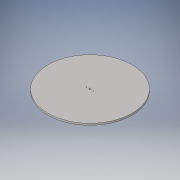
# Autodesk Inventor part: Zoetrope_Top
Saved by Autodesk Inventor 2016 (Build 200138000, 138)
## iProperties
Created: 2019-02-14
Part Number: Zoetrope_Top
Material: Generic
Document SubType Name: Modeling
Designer: student
Density: 1 g/cm^3
Appearance: Default
Author: student
Autodesk Inventor part; units mm, degrees
ref_plane "YZ Plane" through (0, 0, 0) normal (1, 0, 0) x (0, 1, 0)
ref_plane "XZ Plane" through (0, 0, 0) normal (0, 1, 0) x (-1, 0, 0)
ref_plane "XY Plane" through (0, 0, 0) normal (0, 0, 1) x (1, 0, 0)
sketch "Sketch1" plane through (0, 0, 0) normal (0, 1, 0) x (-1, 0, 0)
  circle A0 centre (0, 0) radius 114.3
  line L0 (0, 0) -> (80.8223, -80.8223)
  line L1 (0, 0) -> (114.3, 0)
  line L2 (0, 0) -> (80.8223, 80.8223)
  line L3 (0, 0) -> (114.3, 0) construction
  line L4 (0, 0) -> (-80.8223, -80.8223)
  line L5 (0, 0) -> (114.3, 0) construction
  line L6 (0, 0) -> (-80.8223, 80.8223)
  line L7 (0, 0) -> (114.3, 0) construction
  line L8 (0, 0) -> (114.3, 0) construction
  line L9 (0, 0) -> (114.3, 0) construction
  line L10 (0, 0) -> (114.3, 0) construction
  line L11 (0, 114.3) -> (0, 0)
  line L12 (0, 0) -> (-114.3, 0)
  line L13 (0, 0) -> (0, -114.3)
  line L14 (0, 0) -> (114.3, 0) construction
  circle A1 centre (0, 0) radius 2.2225
  line L15 (0, 0) -> (-9.525, 0)
  circle A2 centre (-9.525, 0) radius 0.9525
  line L16 (0, 0) -> (9.525, 0)
  circle A3 centre (9.525, 0) radius 0.9525
  line L17 (80.8223, -80.8223) -> (53.8815, -53.8815)
  line L18 (0, -114.3) -> (0, -76.2)
  line L19 (0, 0) -> (34.0206, -82.1329) construction
  line L20 (0, 0) -> (101.6, 0) construction
  line L21 (0, 0) -> (-34.0206, 82.1329) construction
  line L22 (0, 0) -> (-34.0206, -82.1329) construction
  line L23 (0, 0) -> (34.0206, 82.1329) construction
  line L24 (0, 0) -> (82.1329, -34.0206) construction
  line L25 (0, 0) -> (-82.1329, 34.0206) construction
  line L26 (0, 0) -> (-82.1329, -34.0206) construction
  line L27 (0, 0) -> (82.1329, 34.0206) construction
  circle A4 centre (0, 0) radius 88.9
  dimension "d0" = 228.6
  dimension "d27" = 177.8
  dimension "d1" = 45
  dimension "d2" = 45
  dimension "d3" = 135
  dimension "d4" = 135
  dimension "d12" = 4.445
  dimension "d13" = 9.525
  dimension "d14" = 1.905
  dimension "d15" = 9.525
  dimension "d16" = 1.905
  dimension "d22" = 67.5
  dimension "d23" = 22.5
  dimension "d24" = 22.5
  dimension "d25" = 22.5
  dimension "d26" = 22.5
  dimension "d28" = 22.5
  dimension "d29" = 22.5
  dimension "d30" = 22.5
  constraints: 56 end point, 8 horizontal, 6 coincident, 5 point on line, 4 equal length, 3 centre point, 1 collinear, 1 perpendicular, 1 vertical, 19 other
  measures "d1" angle of L0 L1
  measures "d2" angle of L3 L2
  measures "d3" angle of L4 L5
  measures "d4" angle of L7 L6
  measures "d12" diameter of A1
  measures "d13" distance of L15.start L15.end
  measures "d14" diameter of A2
  measures "d15" distance of L15.start L16.end
  measures "d16" diameter of A3
  measures "d22" angle of L19 L20
  measures "d23" angle of L16 L24
  measures "d24" angle of L4 L22
  measures "d25" angle of L12 L26
  measures "d26" angle of L16 L27
  measures "d28" angle of L25 L12
  measures "d29" angle of L21 L6
  measures "d30" angle of L23 L11
extrude "Extrusion1" add sketch "Sketch1" along normal blind 4.572 contours L1 A4 L2 A0 | A0 L0 A4 L1 | L2 A4 L11 A0 | A0 L13 A4 L0 | A4 L0 A1 L1 A3 | L1 A3 A1 L2 A4 | L11 A4 L6 A0 | L2 A1 L11 A4 | A0 L4 A4 L13 | A4 L13 A1 L0 | L6 A4 L12 A0 | L11 A1 L6 A4 | A0 L12 A4 L4 | A4 L4 A1 L13 | L6 A1 L12 A2 A4 | A4 L12 A2 A1 L4
body "Solid1"
